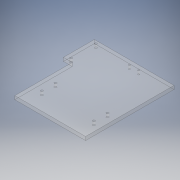
# Autodesk Inventor part: pibot_baseplate
Saved by Autodesk Inventor 2018 (Build 220112000, 112)
## iProperties
Created: 2018-05-04
Part Number: pibot_baseplate
Material: Polycarbonate, Clear
Document SubType Name: Sheet Metal
Designer: mmarkle
Density: 1.2 g/cm^3
Sheet Metal Rule: Default
Appearance: Polycarbonate - Clear
Mass: 78.4023 g
Surface Area: 283.272 cm^2
Volume: 65.3352 cm^3
motor_placement: 1.000 in
Author: mmarkle
Autodesk Inventor part; units mm, degrees
ref_plane "YZ Plane" through (0, 0, 0) normal (1, 0, 0) x (0, 1, 0)
ref_plane "XZ Plane" through (0, 0, 0) normal (0, 1, 0) x (-1, 0, 0)
ref_plane "XY Plane" through (0, 0, 0) normal (0, 0, 1) x (1, 0, 0)
sketch "Sketch1" plane through (0, 0, 0) normal (0, 1, 0) x (-1, 0, 0)
  line L0 (-50.8, 63.5) -> (50.8, 63.5)
  line L1 (50.8, 63.5) -> (50.8, -19.05)
  line L2 (50.8, -63.5) -> (-50.8, -63.5)
  line L3 (-50.8, -63.5) -> (-50.8, 63.5)
  line L4 (-50.8, 63.5) -> (50.8, -63.5) construction
  line L5 (50.8, 63.5) -> (-50.8, -63.5) construction
  line L6 (50.8, -63.5) -> (63.5, -63.5)
  line L7 (63.5, -63.5) -> (63.5, -19.05)
  line L8 (63.5, -19.05) -> (50.8, -19.05)
  line L9 (50.8, -19.05) -> (50.8, -63.5) construction
  point P0 (0, 0)
  point P1 (0, 0)
  dimension "d0" = 101.6
  dimension "d1" = 127
  dimension "d24" = 12.7
  dimension "d25" = 44.45
  measures "d0" distance of L2.start L2.end
  measures "d1" distance of L0.end L2.start
  measures "d24" distance of L1.end L7.end
  measures "d25" distance of L6.end L7.end
extrude "Plate1" add sketch "Sketch1" along normal blind 5.08
sketch "Sketch2" plane through (0, 5.08, 0) normal (0, 1, 0) x (1, 0, 0)
  line L0 (-63.5, 63.5) -> (50.8, 63.5) construction
  line L1 (0, 63.5) -> (0, -63.5) construction
  line L2 (50.8, -63.5) -> (-50.8, -63.5) construction
  line L3 (-50.8, -63.5) -> (-50.8, 19.05) construction
  point P0 (0, 0)
  point P1 (-37.338, -38.1)
  point P2 (-37.338, -18.542)
  point P3 (37.338, -38.1)
  point P4 (37.338, -18.542)
  point P5 (-50.8, 63.5)
  dimension "d5" = 19.558
  dimension "d6" = 13.462
  dimension "d14" = 25.4
  constraints: 2 end point, 2 horizontal alignment, 2 vertical alignment, 1 midpoint, 1 point on line, 1 symmetric about line
  measures "d5" distance of point (-37.338, -38.1) point (-37.338, -18.542)
  measures "d6" distance from line of L3 point (-37.338, -38.1)
  measures "d14" distance from line of point (-37.338, -38.1) L2
hole "Hole1" at (-37.338, 5.08, 38.1) at (-37.338, 5.08, 18.542) at (37.338, 5.08, 38.1) at (37.338, 5.08, 18.542) direction (0, -1, 0) diameter 3.2766 end through all clearance for "Flat Head Machine Screw (82)" size "#4" standard "Ansi Unified Screw Threads"
sketch "Sketch3" plane through (0, 5.08, 0) normal (0, 1, 0) x (1, 0, 0)
  line L0 (0, 0) -> (0, 25.4) construction
  point P0 (-6.604, 56.8607)
  point P1 (6.604, 56.8607)
  dimension "d15" = 25.4
  dimension "d16" = 13.208
  constraints: 2 end point, 1 symmetric about line, 1 vertical
  measures "d15" distance of L0.start L0.end
  measures "d16" distance of point (6.604, 56.861) point (-6.604, 56.861)
hole "Hole2" at (-6.604, 5.08, -56.8607) at (6.604, 5.08, -56.8607) direction (0, -1, 0) diameter 2.286 end through all
sketch "Sketch4" plane through (0, 5.08, 0) normal (0, 1, 0) x (1, 0, 0)
  line L0 (-63.5, 19.05) -> (-63.5, 63.5) projected
  point P0 (0, 0)
  point P1 (-57.15, 23.6543)
  point P2 (-57.15, 59.2143)
  dimension "d26" = 35.56
  dimension "d34" = 6.35
  constraints: 1 vertical alignment
  measures "d26" distance of point (-57.15, 23.654) point (-57.15, 59.214)
  measures "d34" distance from line of L0 point (-57.15, 59.214)
hole "Hole3" at (-57.15, 5.08, -23.6543) at (-57.15, 5.08, -59.2143) direction (0, -1, 0) diameter 3.2766 end through all clearance for "Flat Head Machine Screw (82)" size "#4" standard "Ansi Unified Screw Threads"
equation "\"d14\" = motor_placement"
equation "\"d12\" = Thickness"
equation "\"d22\" = Thickness"
equation "\"d32\" = Thickness"
equation "\"d4\" = Thickness"
equation "\"BendRadius\" = Thickness"
equation "\"BendReliefWidth\" = Thickness"
equation "\"BendReliefDepth\" = 0.5 * Thickness"
equation "\"CornerReliefSize\" = 4 * Thickness"
equation "\"MinimumRemnant\" = 2 * Thickness"
equation "\"TransitionRadius\" = BendRadius"
equation "\"JacobiRadiusSize\" = BendRadius"
equation "\"GapSize\" = Thickness"
equation "\"motor_placement\" = 25.4"
equation "\"Thickness\" = 5.08"
body "Solid1"
